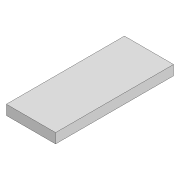
# Autodesk Inventor part: base
Saved by Autodesk Inventor 2020.2 (Build 242310000, 310)
## iProperties
Created: 2020-02-17
Part Number: base
Material: Generic
Document SubType Name: Modeling
Designer: Yash
Density: 1 g/cm^3
Appearance: Default
Author: Yash
Autodesk Inventor part; units mm, degrees
ref_plane "YZ Plane" through (0, 0, 0) normal (1, 0, 0) x (0, 1, 0)
ref_plane "XZ Plane" through (0, 0, 0) normal (0, 1, 0) x (-1, 0, 0)
ref_plane "XY Plane" through (0, 0, 0) normal (0, 0, 1) x (1, 0, 0)
sketch "Sketch1" plane through (0, 0, 0) normal (0, 1, 0) x (-1, 0, 0)
  line L0 (137.2529, 244.1848) -> (87.2529, 244.1848)
  line L1 (87.2529, 244.1848) -> (87.2529, 124.1848)
  line L2 (87.2529, 124.1848) -> (137.2529, 124.1848)
  line L3 (137.2529, 124.1848) -> (137.2529, 244.1848)
  point P0 (0, 0)
  dimension "d0" = 50
  dimension "d1" = 120
  constraints: 8 end point, 2 parallel, 1 horizontal, 1 perpendicular
  measures "d0" distance of L2.end L1.end
  measures "d1" distance of L1.end L0.end
extrude "Extrusion1" add sketch "Sketch1" along normal blind 10
body "Solid1"
